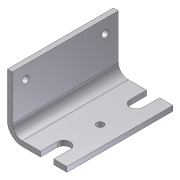
# Autodesk Inventor part: GE-12073
Saved by Autodesk Inventor 2012 (Build 160160000, 160)
## iProperties
Created: 2011-10-01
Part Number: GE-12073
Document SubType Name: Modeling
Designer: dfoster
Density: 1 g/cm^3
Description: Bracket, Backboard
Mass: 47.6165 g
Surface Area: 225.861 cm^2
Volume: 47.6165 cm^3
Material: Default
Title: Bracket, Backboard
Author: dfoster
Autodesk Inventor part; units mm, degrees
ref_plane "YZ Plane" through (0, 0, 0) normal (1, 0, 0) x (0, 1, 0)
ref_plane "XZ Plane" through (0, 0, 0) normal (0, 1, 0) x (-1, 0, 0)
ref_plane "XY Plane" through (0, 0, 0) normal (0, 0, 1) x (1, 0, 0)
sketch "Sketch1" plane through (0, 0, 0) normal (0, 0, 1) x (1, 0, 0)
  line L0 (0, 57.15) -> (0, 14.3002)
  line L1 (14.3002, 0) -> (57.15, 0)
  line L2 (57.15, 0) -> (57.15, 4.7752)
  line L3 (57.15, 4.7752) -> (14.3002, 4.7752)
  line L4 (4.7752, 14.3002) -> (4.7752, 57.15)
  line L5 (4.7752, 57.15) -> (0, 57.15)
  arc A0 (4.7752, 14.3002) -> (14.3002, 4.7752) centre (14.3002, 14.3002) ccw
  arc A1 (0, 14.3002) -> (14.3002, 0) centre (14.3002, 14.3002) ccw
  point P0 (0, 0)
  dimension "d0" = 4.7752
  dimension "d1" = 9.525
  dimension "d2" = 14.3002
  dimension "d3" = 57.15
  constraints: 12 end point, 4 perpendicular, 4 point on circle, 4 tangent, 3 parallel, 2 centre point, 2 point on line, 1 vertical
  measures "d0" distance between parallel lines of L4 L0
  measures "d1" radius of A0
  measures "d2" radius of A1
  measures "d3" distance from line of L2 point (0, 0)
extrude "Extrusion1" add sketch "Sketch1" along normal blind 101.6
hole "Hole1" at (4.7752, 44.45, 88.9) direction (-1, 0, 0) diameter 6.731 end through all
hole "Hole2" at (4.7752, 44.45, 12.7) direction (-1, 0, 0) diameter 6.731 end through all
sketch "Sketch2" plane through (14.3002, 0, 0) normal (0, -1, 0) x (1, 0, 0)
  line L0 (42.8498, 101.6) -> (0, 101.6) projected
  line L1 (0, 0) -> (42.8498, 0) projected
  line L2 (42.8498, 0) -> (42.8498, 101.6) projected
  line L3 (30.1498, 101.6) -> (30.1498, 85.725)
  line L4 (17.4498, 101.6) -> (17.4498, 85.725)
  line L5 (30.1498, 0) -> (30.1498, 15.875)
  line L6 (17.4498, 0) -> (17.4498, 15.875)
  arc A0 (17.4498, 85.725) -> (30.1498, 85.725) centre (23.7998, 85.725) ccw
  arc A1 (30.1498, 15.875) -> (17.4498, 15.875) centre (23.7998, 15.875) ccw
  circle A2 centre (23.7998, 50.8) radius 3.3655
  line L7 (30.1498, 101.6) -> (17.4498, 101.6)
  line L8 (30.1498, 0) -> (17.4498, 0)
  point P0 (-14.3002, 0)
  dimension "d24" = 12.7
  dimension "d25" = 19.05
  dimension "d26" = 15.875
  dimension "d27" = 6.731
  dimension "d28" = 50.8
  dimension "d29" = 19.05
  constraints: 12 end point, 4 parallel, 4 point on circle, 4 tangent, 3 centre point, 3 collinear, 3 equal length, 3 point on line, 1 equal radius
  measures "d24" distance between parallel lines of L3 L4
  measures "d25" distance from line of A0.centre L2
  measures "d26" distance from line of A0.centre L0
  measures "d27" diameter of A2
  measures "d28" distance from line of A2.centre L0
  measures "d29" distance from line of A2.centre L2
extrude "Extrusion2" cut sketch "Sketch2" against normal blind 101.6
equation "\"d2\" = d1 + d0"
equation "\"d29\" = d25"
body "Solid1"
